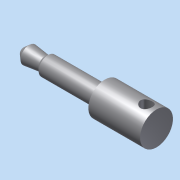
# Autodesk Inventor part: safe_rbf
Saved by Autodesk Inventor 2014 (Build 180170000, 170)
## iProperties
Created: 2013-06-06
Part Number: safe_rbf
Document SubType Name: Modeling
Designer: Robert Davis
Density: 1 g/cm^3
Description: SAFE/ARM RBF
Material: Generic
Appearance: Default
Author: Robert Davis
Autodesk Inventor part; units mm, degrees
ref_plane "YZ Plane" through (0, 0, 0) normal (1, 0, 0) x (0, 1, 0)
ref_plane "XZ Plane" through (0, 0, 0) normal (0, 1, 0) x (-1, 0, 0)
ref_plane "XY Plane" through (0, 0, 0) normal (0, 0, 1) x (1, 0, 0)
sketch "Sketch1" plane through (0, 0, 0) normal (0, 0, 1) x (1, 0, 0)
  line L0 (0, 0) -> (25.9627, 0)
  line L1 (0, 0) -> (0, 0.495)
  line L2 (0, 0.495) -> (0.75, 1.155)
  line L3 (0.75, 1.155) -> (2.9, 0.9)
  line L4 (2.9, 0.9) -> (3.3, 1.25)
  line L5 (3.3, 1.25) -> (11, 1.25)
  line L6 (11, 1.25) -> (11, 0)
  line L7 (11, 0) -> (0, 0)
  dimension "d0" = 0.99
  dimension "d1" = 2.5
  dimension "d2" = 2.31
  dimension "d3" = 0.75
  dimension "d4" = 1.8
  dimension "d5" = 2.9
  dimension "d6" = 3.3
  dimension "d7" = 11
  constraints: 16 end point, 3 horizontal, 2 vertical, 1 coincident
  measures "d0" diameter of L1.end L0
  measures "d1" diameter of L5 L0
  measures "d2" diameter of L2.end L0
  measures "d3" distance from line of L2.end L1
  measures "d4" diameter of L3.end L0
  measures "d5" distance from line of L3.end L1
  measures "d6" distance from line of L1 L4.end
  measures "d7" distance between parallel lines of L6 L1
revolve "Revolution1" add sketch "Sketch1" angle 360 about axis through (0, 0, 0) along (1, 0, 0)
sketch "Sketch2" plane through (11, 0, 0) normal (1, 0, 0) x (0, 0, -1)
  circle A0 centre (0, 0) radius 1.25 projected
  circle A1 centre (0, 0) radius 2.225
  dimension "d9" = 4.45
  constraints: 1 centre point, 1 coincident
  measures "d9" diameter of A1
extrude "Extrusion1" add sketch "Sketch2" along normal blind 7 contours A0 | A1
sketch "Sketch3" plane through (0, 0, 0) normal (0, 0, 1) x (1, 0, 0)
  circle A0 centre (16.6444, 0) radius 0.7937
  line L0 (18, 2.225) -> (18, -2.225) projected
  point P0 (0, 0)
  dimension "d12" = 1.5875
  dimension "d13" = 1.3556
  constraints: 1 centre point
  measures "d12" diameter of A0
  measures "d13" distance from line of L0 A0.centre
extrude "Extrusion2" cut sketch "Sketch3" along normal through all both and the other way through all
body "Solid1"
